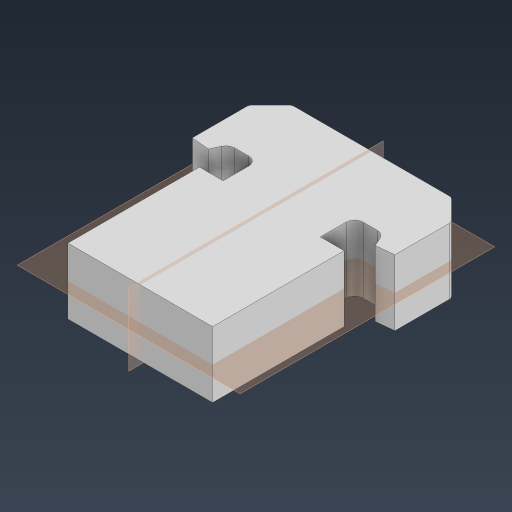
# Autodesk Inventor part: буль
Saved by Autodesk Inventor 2023.2 (Build 272271030, 271C)
## iProperties
Created: 2025-08-26
Part Number: буль
Material: Типовые
Document SubType Name: Modeling
Designer: Олег Коноваленко
Density: 1 g/cm^3
Appearance: По умолчанию
Author: Олег Коноваленко
Autodesk Inventor part; units mm, degrees
ref_plane "XY Plane" through (0, 0, 0) normal (0, 0, 1) x (1, 0, 0)
sketch "Эскиз1" plane through (0, 0, 0) normal (0, 1, 0) x (-1, 0, 0)
  line L0 (5.5, 5) -> (-5.5, 5)
  line L1 (-5.5, 5) -> (-5.5, -5)
  line L2 (-5.5, -5) -> (5.5, -5)
  line L3 (5.5, -5) -> (5.5, 5)
  line L4 (5.5, 5) -> (-5.5, -5) construction
  line L5 (-5.5, 5) -> (5.5, -5) construction
  point P0 (0, 0)
  dimension "d0" = 11
  dimension "d1" = 10
  constraints: 12 end point, 2 midpoint, 2 parallel, 1 horizontal, 1 perpendicular
  measures "d0" distance of L1.end L2.end
  measures "d1" distance of L0.end L1.end
extrude "Выдавливание1" add sketch "Эскиз1" along normal mid plane 5
sketch "Эскиз3" plane through (0, 2.5, 0) normal (0, 1, 0) x (1, 0, 0)
  arc A0 (-5.15, 5) -> (-4.9, 5.25) centre (-5.15, 5.25) ccw projected
  line L0 (-4.9, 5.8) -> (-4.9, 5.25) projected
  line L1 (-4.35, 5.8) -> (-4.9, 5.8) projected
  arc A1 (-4.35, 5.8) -> (-4.1, 6.05) centre (-4.35, 6.05) ccw projected
  line L2 (-4.1, 6.95) -> (-4.1, 6.05) projected
  arc A2 (-4.1, 6.95) -> (-4.35, 7.2) centre (-4.35, 6.95) ccw projected
  line L3 (-5.439, 7.2) -> (-4.35, 7.2) projected
  arc A3 (-5.439, 7.2) -> (-5.6666, 7.0535) centre (-5.439, 6.95) ccw projected
  line L4 (-6.0258, 6.2631) -> (-5.6666, 7.0535) projected
  arc A4 (-6.2783, 6.1178) -> (-6.0258, 6.2631) centre (-6.2534, 6.3666) ccw projected
  line L5 (-7.8749, 6.2775) -> (-6.2783, 6.1178) projected
  arc A5 (-8.1, 6.5262) -> (-7.8749, 6.2775) centre (-7.85, 6.5262) ccw projected
  line L6 (-8.1, 10.8115) -> (-8.1, 6.5262) projected
  arc A6 (-7.8803, 11.3419) -> (-8.1, 10.8115) centre (-7.35, 10.8115) ccw projected
  arc A7 (8.1, 10.8115) -> (7.8803, 11.3419) centre (7.35, 10.8115) ccw projected
  line L7 (8.1, 6.5262) -> (8.1, 10.8115) projected
  arc A8 (7.8749, 6.2775) -> (8.1, 6.5262) centre (7.85, 6.5262) ccw projected
  line L8 (6.2783, 6.1178) -> (7.8749, 6.2775) projected
  arc A9 (6.0258, 6.2631) -> (6.2783, 6.1178) centre (6.2534, 6.3666) ccw projected
  line L9 (5.6666, 7.0535) -> (6.0258, 6.2631) projected
  arc A10 (5.6666, 7.0535) -> (5.439, 7.2) centre (5.439, 6.95) ccw projected
  line L10 (4.35, 7.2) -> (5.439, 7.2) projected
  arc A11 (4.35, 7.2) -> (4.1, 6.95) centre (4.35, 6.95) ccw projected
  line L11 (4.1, 6.05) -> (4.1, 6.95) projected
  arc A12 (4.1, 6.05) -> (4.35, 5.8) centre (4.35, 6.05) ccw projected
  line L12 (4.9, 5.8) -> (4.35, 5.8) projected
  line L13 (4.9, 5.25) -> (4.9, 5.8) projected
  arc A13 (4.9, 5.25) -> (5.15, 5) centre (5.15, 5.25) ccw projected
  line L14 (7.8803, 11.3419) -> (6.4419, 12.7803) projected
  arc A14 (6.4419, 12.7803) -> (5.9115, 13) centre (5.9115, 12.25) ccw projected
  line L15 (5.9115, 13) -> (0.4906, 13) projected
  line L16 (-0.4906, 13) -> (-5.9115, 13) projected
  arc A15 (-5.9115, 13) -> (-6.4419, 12.7803) centre (-5.9115, 12.25) ccw projected
  line L17 (-6.4419, 12.7803) -> (-7.8803, 11.3419) projected
  line L18 (0.4906, 13) -> (-0.4906, 13)
  line L19 (-3.7, 6.05) -> (-3.7, 6.95)
  arc A16 (-3.7, 6.95) -> (-4.35, 7.6) centre (-4.35, 6.95) ccw
  line L20 (-4.35, 7.6) -> (-5.439, 7.6)
  arc A17 (-5.439, 7.6) -> (-6.0308, 7.219) centre (-5.439, 6.95) ccw
  line L21 (-6.0308, 7.219) -> (-6.3455, 6.5265)
  line L22 (-6.3455, 6.5265) -> (-7.7, 6.662)
  line L23 (-7.7, 6.662) -> (-7.7, 10.8115)
  arc A18 (-7.5975, 11.059) -> (-7.7, 10.8115) centre (-7.35, 10.8115) ccw
  line L24 (-7.5975, 11.059) -> (-6.159, 12.4975)
  arc A19 (-5.9115, 12.6) -> (-6.159, 12.4975) centre (-5.9115, 12.25) ccw
  line L25 (-5.9115, 12.6) -> (-0.4906, 12.6)
  line L26 (-0.4906, 12.6) -> (0.4906, 12.6)
  line L27 (0.4906, 12.6) -> (5.9115, 12.6)
  arc A20 (6.159, 12.4975) -> (5.9115, 12.6) centre (5.9115, 12.25) ccw
  line L28 (6.159, 12.4975) -> (7.5975, 11.059)
  arc A21 (7.7, 10.8115) -> (7.5975, 11.059) centre (7.35, 10.8115) ccw
  line L29 (7.7, 10.8115) -> (7.7, 6.662)
  line L30 (7.7, 6.662) -> (6.3455, 6.5265)
  line L31 (6.3455, 6.5265) -> (6.0308, 7.219)
  arc A22 (6.0308, 7.219) -> (5.439, 7.6) centre (5.439, 6.95) ccw
  line L32 (5.439, 7.6) -> (4.35, 7.6)
  arc A23 (4.35, 7.6) -> (3.7, 6.95) centre (4.35, 6.95) ccw
  line L33 (3.7, 6.95) -> (3.7, 6.1534)
  line L34 (3.7, 6.1534) -> (3.7, 5)
  line L35 (5.5, 5) -> (-5.5, 5) projected
  line L36 (-3.7, 6.05) -> (-3.7, 5)
  point P0 (0, 0)
  point P1 (-4.9967, 19.8192)
  dimension "d6" = 0.4
  constraints: 36 end point, 16 point on circle, 8 centre point, 2 perpendicular, 2 point on line, 1 horizontal, 22 other
  measures "d6" distance between parallel lines of L27 L15
extrude "Выдавливание3" add sketch "Эскиз3" against normal up to surface (5 mm away) contours L36 L19 A16 L20 A17 L21 L22 L23 A18 L24 A19 L25 L26 L27 A20 L28 A21 L29 L30 L31 A22 L32 A23 L33 L34 L35
